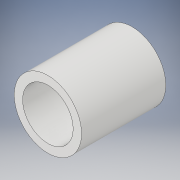
# Autodesk Inventor part: CAR_39_1inchSpacers
Saved by Autodesk Inventor 2018 (Build 220112000, 112)
## iProperties
Created: 2020-02-09
Part Number: CAR_39_1inchSpacers
Material: PVC-Piping
Document SubType Name: Modeling
Designer: jd2
Density: 1.4 g/cm^3
Appearance: Smooth - White
Author: jd2
Autodesk Inventor part; units mm, degrees
ref_plane "YZ Plane" through (0, 0, 0) normal (1, 0, 0) x (0, 1, 0)
ref_plane "XZ Plane" through (0, 0, 0) normal (0, 1, 0) x (-1, 0, 0)
ref_plane "XY Plane" through (0, 0, 0) normal (0, 0, 1) x (1, 0, 0)
sketch "Sketch1" plane through (0, 0, 0) normal (0, 0, 1) x (1, 0, 0)
  circle A0 centre (0, 0) radius 7.62
  circle A1 centre (0, 0) radius 10.16
  dimension "d0" = 15.24
  dimension "d1" = 2.54
  constraints: 2 centre point, 1 coincident
  measures "d0" diameter of A0
  measures "d1" radial gap between concentric circles of A0 A1
extrude "Extrusion1" add sketch "Sketch1" along normal blind 25.4
body "Solid1"
